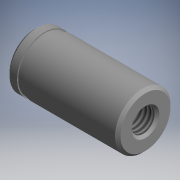
# Autodesk Inventor part: SSFRBF-D10-L20-M5-U3
Saved by Autodesk Inventor 2017.3 (Build 213256000, 256)
## iProperties
Part Number: SSFRBF-D10-L20-M5-U3
Material: Generic
Catalog Web Link: www.cadenas.de
Description: NSFR_ _, SFR_ _, PSFR_ _, SSFR_ _-Rotary Shafts - Ends Shape Combination Type
Vendor: MISUMI
Document SubType Name: Modeling
Designer: partserver
Manufacturer: MISUMI
Mass: 1.36416 g
Surface Area: 9.55552 cm^2
Volume: 1.36416 cm^3
Density: 1 g/cm^3
Appearance: PSOLRGB-175-175-175
Category: PARTsolutions
Company: MISUMI
Title: SSFRBF-D10-L20-M5-U3
Author: Cadenas PARTsolutions
Comments: Rotary Shafts - Ends Shape Combination Type
PSOL_IDENT_0: {$CADENAS_DATA\23d-libs\misumi\metric\11_rotary_shafts\psfrbf.prj},506 {VTYP=3D},{NB=SSFRBF-D10-L20-
PSOL_IDENT_1: M5-U3},{LINA=SSFRBF-D10-L20-M5-U3},{NN=NSFR_ _, SFR_ _, PSFR_ _, SSFR_ _},{DATE=27.07.2021 05:05:26}
PSOL_IDENT_2: ,{GEOMDATE=14.12.2020 07:15:28},{VERSION=},{LINEID=10},{WBVAR=MAT,ST,LES,RES,D,ALT1,L,ALT9,ALT13,F,B
PSOL_IDENT_3: ,H,PMC,CM,P,M,R,ALT18,T,S,U,QNC,CN,Q,N,W,ALT2,KC,A,WKC,CALT2,K,E,ALT8,PKC,ALT14,QKC,ALT3,FC,GALT3,WF
PSOL_IDENT_4: C,J,WALT3,V,ALT4,SFC,SG,AG,ALT5,UC,ALT7,SC,ALT12,ALT15},{WBNUMERIC=D,L,F,B,H,PMC,CM,P,M,R,T,S,U,QNC,
PSOL_IDENT_5: CN,Q,N,W,KC,A,WKC,CALT2,K,E,PKC,QKC,FC,GALT3,WFC,J,WALT3,V,SFC,SG,AG,UC,SC}  {NB=SSFRBF-D10-L20-M5-U
PSOL_IDENT_6: 3},{LINA=SSFRBF-D10-L20-M5-U3},{KT=DUMMY},{PN=SSFRBF-D10-L20-M5-U3},{TS=NSFR_ _, SFR_ _, PSFR_ _, SS
PSOL_IDENT_7: FR_ _},{MAT=SUS304},{MATALG= 'S45C','1045 Carbon Steel','SUS304','304 Stainless Steel' },{ST=},{STAL
PSOL_IDENT_8: G= '','-' },{TYPE=SSFR},{LES=B},{LESALG= 'A','A','B','B','C','C','D','D','E','E','F','F','G','G','H'
PSOL_IDENT_9: ,'H','J','J' },{RES=F},{RESALG= 'A','A','B','B','C','C','D','D','E','E','F','F','G','G','H','H','J','
PSOL_IDENT_10: J' },{PNL=-M5},{PNR=-U3},{D=10},{DALG=[6:26/1],[28:30/1],[32],[35],[40],[45],[50]},{DJMIN=15},{YMAX=
PSOL_IDENT_11: 500},{Y=20},{ALT1=},{ALT1ALG= '','w/o LKC (Changes L Tolerance)','-LKC','with LKC (Changes L Toleran
PSOL_IDENT_12: ce)' },{L=20.0},{LALG=[20:500/0.1]},{LMIN=20},{LMAX=500},{CIFSFL=0},{CIFSFR=0},{ALT9=},{ALT9ALG= '','
PSOL_IDENT_13: N/A' },{ALT13=},{ALT13ALG= '','N/A' },{F=0.0},{FALG=[0]},{FMIN=2},{FCMIN=5},{FCMINALG=2},{CIFFCMINAL
PSOL_IDENT_14: G=4},{FCPICTHALG=0.7},{FGMIN=4},{FHMIN=2},{FJMIN=3},{CIFFMIN=2},{FMAX=45},{B=0},{BALG=[0]},{BMIN=2},
PSOL_IDENT_15: {CIFBCMIN=4},{CIFBCMINALG=4},{BCPICTHALG=0.7},{BMAX=-3},{CIFBD=8},{H=0},{HALG=[0]},{HFALG=[0]},{HFMI
PSOL_IDENT_16: N=3},{HFMAX=15},{HGALG=[0]},{HGMIN=2},{HGMAX=-2},{PMC=0},{PMCALG=0},{PMCPMIN=0},{PMCPMINALG=3},{PMCD
PSOL_IDENT_17: MIN=4},{PMCBMIN=0},{PMCBMINALG=3},{PMCMIN=4},{PMCDMAX=9},{PMCDMAXALG=8},{PMCMAX=8},{CM=0},{CMALG=0},
PSOL_IDENT_18: {CMDMIN=4},{CMBMIN=0},{CMFMIN=0},{CMMIN=4},{CMMINALG=4},{CMMAX=9},{CMMAXALG=8},{P=0},{PALG=[0]},{PMI
PSOL_IDENT_19: N=4},{PMINALG=4.000},{PMIND=4},{PMINF=0},{PEMIN=5},{PMAX=9},{PMAXH=9},{PGMAX=9},{PGMAXALG=9},{PGALG=
PSOL_IDENT_20: [4:9/1]},{M=5},{MALG=3,4,5,6},{BMALG=3,4,5,6},{BEMALG=3,4,5,6},{BETMAX=45},{BFMALG=3,4,5,6},{BBMALG=
PSOL_IDENT_21: 3,4,5},{CIFBM=0},{EMALG=0},{EBMALG=0},{EEMALG=0},{EETMAX=45},{HBMALG=3,4,5,6},{HEMALG=0},{JMALG=0},{
PSOL_IDENT_22: CIFJM=0},{JMMAX=2},{JMMAXALG=2},{PITCHM=0.8},{PITCHPMC=0},{ITM=2},{ML=15},{DDL=0},{DDP=0},{MML=0},{H
PSOL_IDENT_23: LL=0},{R=0},{RALG=[0]},{RMIN=8},{RMAX=1},{JMDIA=5},{ALT18=},{ALT18ALG= '','N/A' },{T=0.0},{TALG=[0]}
PSOL_IDENT_24: ,{TMIN=2},{TCMIN=5},{TCMINALG=2},{CIFTCMINALG=4},{TCPICTHALG=0.7},{TGMIN=4},{THEMIN=2},{TJEMIN=3},{C
PSOL_IDENT_25: IFTMIN=2},{CIFTMIN1=2},{TMAX=45.000},{TMAXBE=500},{TMAXEE=500},{S=0},{SALG=[0]},{SMIN=2},{CIFSCMIN=4
PSOL_IDENT_26: },{CIFSCMINALG=4},{SCPICTHALG=0.7},{SMAX=-3},{CIFSD=8},{U=3},{UALG=[3:17/1]},{UFALG=[3:17/1]},{UFMIN=
PSOL_IDENT_27: 3},{UFMAX=17},{UGALG=[0]},{UGMIN=2},{UGMAX=-2},{QNC=0},{QNCALG=0},{QNCQMIN=0},{QNCQMINALG=3},{QNCDMI
PSOL_IDENT_28: N=4},{QNCSMIN=0},{QNCSMINALG=3},{QNCMIN=4},{QNCDMAX=9},{QNCDMAXALG=8},{QNCMAX=8},{CN=0},{CNALG=0},{C
PSOL_IDENT_29: NDMIN=4},{CNSMIN=0},{CNTMIN=0},{CNMIN=4},{CNMINALG=4},{CNMAX=9},{CNMAXALG=8},{Q=0},{QALG=[0]},{QMIN=
PSOL_IDENT_30: 4},{QMINALG=4.000},{QMIND=4},{QMINT=0},{QEMIN=7},{QBEMIN=7},{QMAX=9},{QMAXU=10},{QGMAX=9},{QGMAXALG=
PSOL_IDENT_31: 9},{QGALG=[4:9/1]},{N=0},{NALG=[0]},{CIFBN=10},{BANALG=3,4,5,6},{BBNALG=5},{BBNMAX=0},{BBNALGMEQN=5}
PSOL_IDENT_32: ,{BBNALGMGTN=0},{BBNALGMLTN=0},{BENALG=},{BENMAX=0},{BENALGMEQN=5},{BENALGMGTN=0},{BENALGMLTN=0},{BF
PSOL_IDENT_33: NALG=3,4,5,6},{BJNALG=0},{ENALG=0},{EBNALG=5},{EBNMAX=0},{EBNALGMEQN=5},{EBNALGMGTN=0},{EBNALGMLTN=0
PSOL_IDENT_34: },{EENALG=},{EENMAX=0},{EENALGMEQN=5},{EENALGMGTN=0},{EENALGMLTN=0},{HBNALG=3,4,5,6},{HENALG=0},{JNA
PSOL_IDENT_35: LG=0},{CIFJN=17},{JNJALG=4},{JNMAX=1},{JNMAXALG=1},{PITCHN=0},{PITCHQNC=0},{ITN=0},{NL=0},{DDR=9.6},
PSOL_IDENT_36: {DDF=9.6},{DDQ=0},{MMR=1.15},{BB=0},{BBDIA=0},{BBNML=4.134},{HH=0},{HLR=0},{W=0},{WALG=[0]},{WMIN=3}
PSOL_IDENT_37: ,{WMAX=6},{JNDIA=0},{C=0.5},{PNALT=},{ALT2=},{ALT2ALG= '', 'w/o Key Grooves','KC','with KC (Key Groo
PSOL_IDENT_38: ve)','WKC','with WKC (Two Key Grooves)','KCWKC','with KC + WKC (Three Key Grooves)' },{ALT2PN=},{KC=
PSOL_IDENT_39: 0.0},{KCALG=[0]},{KCMIN=0},{KCMAX1=17},{KCMAX2=11},{A=0.0},{AALG=[0]},{AMIN=3},{AMAX1=20},{AMAX2=14}
PSOL_IDENT_40: ,{WKC=0.0},{WKCALG=[0]},{WKCMIN1=0},{WKCMIN2=0},{WKCMAX1=14},{CALT2=0.0},{CALT2ALG=[0]},{CALT2MIN=3}
PSOL_IDENT_41: ,{CALT2MAX1=17},{K=0.0},{KALG=[0]},{KMIN1=0},{KMAX1=17},{E=0.0},{EALG=[0]},{EMIN=3},{EMAX=20},{BBALT
PSOL_IDENT_42: 2=3},{CIFKC=0},{CIFWKC=0},{CIFK=0},{CIKC=0},{TTALT2=1.8},{CIFKG=0},{KGMIN1=0},{KGMIN2=0},{KGMIN3=0},
PSOL_IDENT_43: {KGMAX1=0},{KGMAX2=0},{KGMAX3=0},{CIFKGC=0},{CIFKG1=1},{CIFKG2=0},{CIFKG3=0},{CIFKGP=1},{CIFKGQ=0},{
PSOL_IDENT_44: PCUT3D=0},{QCUT3D=0},{ALT8=},{ALT8ALG= '','N/A' },{ALT8PN=},{PKC=0.0},{PKCALG=[0]},{PKCMIN=0},{PKCMA
PSOL_IDENT_45: X=0},{BBALT8=0},{TTALT8=0},{CIFPKC=0},{TPKC=0},{ALT14=},{ALT14ALG= '','N/A' },{ALT14PN=},{QKC=0.0},{
PSOL_IDENT_46: QKCALG=[0]},{QKCMIN=0},{QKCMAX=0},{BBALT14=0},{TTALT14=0},{CIFQKC=0},{TQKC=0},{ALT3=},{ALT3ALG= '', '
PSOL_IDENT_47: w/o Set Screw Flat','FC','with FC (Adds a Set Screw Flat)','WFC','with WFC (Adds Two Set Screw Flats
PSOL_IDENT_48: )','FCWFC','with FC + WFC (Adds Three Set Screw Flats)' },{ALT3PN=},{FC=0},{FCALG=[0]},{FCMINALT3=0}
PSOL_IDENT_49: ,{FCMAXALT3=19},{GALT3=0},{GALT3ALG=[0]},{GALT3MIN=1},{GALT3MAX=20},{GALT3MAX2=14},{GALT3MAX3=17},{W
PSOL_IDENT_50: FC=0},{WFCALG=[0]},{WFCMIN=0},{WFCMIN2=2},{WFCMAX=16},{WFCMAX2=-3},{WFCMAX3=-4},{J=0},{JALG=[0]},{JM
PSOL_IDENT_51: IN=1},{JMAX=17},{JMAX2=-2},{JMAX3=-5},{WALT3=0},{WALT3ALG=[0]},{WALT3MIN=0},{WALT3MIN2=22},{WALT3MAX=
PSOL_IDENT_52: 17},{WALT3MAX2=17},{V=0},{VALG=[0]},{VMIN=1},{VMAX=18},{VMAX2=18},{CIFFC=0},{ALT4=},{ALT4ALG= '','w/
PSOL_IDENT_53: o SFC (2 Set Screw Flats (Angle Specified))','SFC','with SFC (2 Set Screw Flats (Angle Specified))'
PSOL_IDENT_54: },{ALT4PN=},{SFC=0},{SFCALG=[0]},{SFCMIN=0},{SFCMAX=19},{SG=0},{SGALG=[0]},{SGMIN=1},{SGMAX=20},{AG=
PSOL_IDENT_55: 0},{AGALG=[0]},{CIFSFC=0},{HHALT34=0},{ALT5=},{ALT5ALG= '', 'w/o UC (Slit Cam Groove)', 'UC', 'with
PSOL_IDENT_56: UC (Slit Cam Groove)'},{ALT5PN=},{UC=0},{UCALG=[0]},{UCMIN=1},{UCMAX=14},{DDALT5=0},{LL1=0},{ALT7=},
PSOL_IDENT_57: {ALT7ALG= '','w/o SC (Wrench Flats)','SC','with SC (Wrench Flats)' },{ALT7PN=},{SC=0},{SCALG=[0]},{S
PSOL_IDENT_58: CMIN=0},{SCMAX=12},{WALT7=0},{LL2=0},{LL2ALG=8},{CIFSC=0},{ALT12=},{ALT12ALG= '','N/A' },{ALT12PN=},
PSOL_IDENT_59: {PC=0},{Z1=0},{Z11=0},{ALT15=},{ALT15ALG= '','N/A' },{ALT15PN=},{QC=0},{QZ1=0},{QZ11=0},{CIFCALC1=0}
PSOL_IDENT_60: ,{CIFCALC2=0},{CIFCALC3=0},{ERRORPN=},{ERRORMALT2=OK},{ERRORMALT3=OK},{ERRORMALT4=OK},{ERRORMALT5=OK
PSOL_IDENT_61: },{ERRORMALT7=OK},{ERRORRALT2=OK},{ERRORRALT3=OK},{ERRORRALT4=OK},{ERRORRALT5=OK},{ERRORRALT7=OK},{E
PSOL_IDENT_62: RRORRGALT2=OK},{ERRORHALT2=OK},{ERRORHALT3=OK},{ERRORHALT4=OK},{ERRORHALT5=OK},{ERRORHALT7=OK},{ERRO
PSOL_IDENT_63: RJALT2=OK},{ERRORJALT3=OK},{ERRORJALT4=OK},{ERRORJALT5=OK},{ERRORJALT7=OK},{ERRORALT23=OK},{ERRORALT
PSOL_IDENT_64: 24=OK},{ERRORALT25=OK},{ERRORALT27=OK},{ERRORALT28=OK},{ERRORALT214=OK},{ERRORALT34=OK},{ERRORALT35=
PSOL_IDENT_65: OK},{ERRORALT37=OK},{ERRORALT45=OK},{ERRORALT47=OK},{ERRORALT57=OK},{ERRORALT812=OK},{ERRORALT1415=O
PSOL_IDENT_66: K},{ERROREMALT8=OK},{ERRORENALT14=OK},{CIFMN3D=0},{ERRORML=15},{ERRORNL=0},{ML3D=15},{NL3D=0}
NB: SSFRBF-D10-L20-M5-U3
NN: NSFR_ _, SFR_ _, PSFR_ _, SSFR_ _
NT: Rotary Shafts - Ends Shape Combination Type
NBSYN: $PN.
LINA: SSFRBF-D10-L20-M5-U3
CATALOG: Misumi
PN: SSFRBF-D10-L20-M5-U3
TS: NSFR_ _, SFR_ _, PSFR_ _, SSFR_ _
MAT: 304 Stainless Steel
ST: -
LES: B
RES: F
D: 10
ALT1: w/o LKC (Changes L Tolerance)
L: 20
ALT9: N/A
ALT13: N/A
F: 0
B: 0
H: 0
PMC: 0
CM: 0
P: 0
M: 5
R: 0
ALT18: N/A
T: 0
S: 0
U: 3
QNC: 0
CN: 0
Q: 0
N: 0
W: 0
C: 0.5
ALT2: w/o Key Grooves
KC: 0
A: 0
WKC: 0
CALT2: 0
K: 0
E: 0
ALT8: N/A
PKC: 0
ALT14: N/A
QKC: 0
ALT3: w/o Set Screw Flat
FC: 0
GALT3: 0
WFC: 0
J: 0
WALT3: 0
V: 0
ALT4: w/o SFC (2 Set Screw Flats (Angle Specified))
SFC: 0
SG: 0
AG: 0
HHALT34: 0
ALT5: w/o UC (Slit Cam Groove)
UC: 0
DDALT5: 0
LL1: 0
ALT7: w/o SC (Wrench Flats)
SC: 0
WALT7: 0
LL2: 0
ALT12: N/A
ALT15: N/A
SUPPLIER: MISUMI
ARTICLENO: SSFRBF-D10-L20-M5-U3
BOMINFO: SSFRBF-D10-L20-M5-U3
CREATOR: CADENAS GmbH
Autodesk Inventor part; units mm, degrees
sketch "Sketch_1" plane through (0, 0, 0) normal (0, 0, 1) x (1, 0, 0)
  line L0 (20, 0) -> (0, 0)
  line L1 (0, 0) -> (0, 4.5)
  line L2 (0, 4.5) -> (0.5, 5)
  line L3 (0.5, 5) -> (19.5, 5)
  line L4 (19.5, 5) -> (20, 4.5)
  line L5 (20, 4.5) -> (20, 0)
  line L6 (20, 0) -> (0, 0)
  constraints: 14 end point
revolve "Revolution1" add sketch "Sketch_1" angle 360 about axis through (20, 0, 0) along (1, 0, 0)
sketch "Sketch2" plane through (0, 0, 0) normal (-1, 0, 0) x (0, 0, 1)
  point P0 (0, 0)
hole "Hole1" at (0, 0, 0) direction (1, 0, 0) diameter 4.134 depth 13.8066 tip angle 120 countersink diameter 5 countersink angle 90 thread size "M5x0.8" class "6H" standard "ISO Metric profile"
sketch "Sketch_20" plane through (0, 0, 0) normal (0, 0, 1) x (1, 0, 0)
  line L0 (20, 0) -> (-20, 0)
  line L1 (17, 9.6) -> (17, 4.8)
  line L2 (17, 4.8) -> (18.15, 4.8)
  line L3 (18.15, 4.8) -> (18.15, 9.6)
  line L4 (18.15, 9.6) -> (17, 9.6)
  constraints: 10 end point
revolve "Revolution2" cut sketch "Sketch_20" angle 360 about axis through (20, 0, 0) along (1, 0, 0)
ref_plane "to_ring_F_R_XY" through (17.575, 0, 0) normal (1, 0, 0) x (0, 0, -1)
ref_plane "to_ring_F_R_YZ" through (17.575, 0, 0) normal (0, 0, -1) x (0, 1, 0)
ref_plane "to_ring_F_R_ZX" through (17.575, 0, 0) normal (0, 1, 0) x (1, 0, 0)
body "Solid1"
